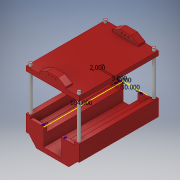
# Autodesk Inventor part: Gondola Shape
Saved by Autodesk Inventor 2018 (Build 220112000, 112)
## iProperties
Created: 2018-01-19
Part Number: Gondola Shape
Material: Steel
Document SubType Name: Modeling
Designer: Joey
Density: 7.85 g/cm^3
Appearance: Red
Author: Joey
Autodesk Inventor part; units mm, degrees
ref_plane "YZ Plane" through (0, 0, 0) normal (1, 0, 0) x (0, 1, 0)
ref_plane "XZ Plane" through (0, 0, 0) normal (0, 1, 0) x (-1, 0, 0)
ref_plane "XY Plane" through (0, 0, 0) normal (0, 0, 1) x (1, 0, 0)
sketch "Sketch1" plane through (0, 0, 0) normal (0, 0, 1) x (1, 0, 0)
  line L0 (0, 3431.8221) -> (1930.4, 3431.8221) construction
  line L1 (1930.4, 3431.8221) -> (1930.4, 0) construction
  line L2 (1930.4, 0) -> (0, 0) construction
  line L3 (0, 0) -> (0, 3431.8221) construction
  line L4 (50.8, 812.8) -> (150.6424, 812.8)
  line L5 (150.6424, 812.8) -> (406.4, 508)
  line L6 (406.4, 508) -> (1524, 508)
  line L7 (1524, 508) -> (1779.7576, 812.8)
  line L8 (1779.7576, 812.8) -> (1879.6, 812.8)
  line L9 (1879.6, 812.8) -> (1879.6, 1371.6)
  line L10 (1879.6, 1371.6) -> (1727.2, 1371.6)
  line L11 (50.8, 1371.6) -> (50.8, 812.8)
  line L12 (203.2, 1371.6) -> (203.2, 1270)
  line L13 (203.2, 1270) -> (660.4, 1270)
  line L14 (660.4, 1270) -> (660.4, 660.4)
  line L15 (660.4, 660.4) -> (1270, 660.4)
  line L16 (1270, 660.4) -> (1270, 1270)
  line L17 (1270, 1270) -> (1727.2, 1270)
  line L18 (1727.2, 1270) -> (1727.2, 1371.6)
  line L19 (203.2, 1371.6) -> (50.8, 1371.6)
  dimension "d9" = 130
  dimension "d27" = 558.8
  dimension "d29" = 1828.8
  dimension "d30" = 1930.4
  dimension "d37" = 101.6
  dimension "d46" = 508
  dimension "d47" = 50.8
  dimension "d51" = 152.4
  dimension "d68" = 1117.6
  dimension "d69" = 304.8
  dimension "d74" = 609.6
  dimension "d77" = 609.6
  constraints: 32 end point, 12 perpendicular, 5 equal length, 4 horizontal, 2 vertical, 1 coincident, 1 collinear, 1 point on line, 2 other
  measures "d9" angle of L5 L4
  measures "d27" distance of L8.end L9.end
  measures "d29" distance between parallel lines of L9 L11
  measures "d30" distance of L1.end L2.end
  measures "d37" distance of L17.end L10.end
  measures "d46" distance from line of L6 point (0, 0)
  measures "d47" distance between parallel lines of L3 L11
  measures "d51" distance of L12.start L11.start
  measures "d68" distance of L5.end L6.end
  measures "d69" distance between parallel lines of L4 L6
  measures "d74" distance of L14.end L15.end
  measures "d77" distance of L13.end L14.end
extrude "Extrusion1" add sketch "Sketch1" along normal mid plane 2743.2
sketch "Sketch2" plane through (203.2, 1270, -1371.6) normal (0, 1, 0) x (1, 0, 0)
  line L0 (0, 0) -> (457.2, 0) construction
  line L1 (0, 0) -> (0, -2743.2) construction
  line L2 (457.2, -2743.2) -> (0, -2743.2) construction
  line L3 (457.2, 0) -> (457.2, -2743.2) construction
  line L4 (1066.8, 0) -> (1524, 0) construction
  line L5 (1066.8, 0) -> (1066.8, -2743.2) construction
  line L6 (1524, -2743.2) -> (1066.8, -2743.2) construction
  line L7 (1524, 0) -> (1524, -2743.2) construction
  line L8 (457.2, -2641.6) -> (0, -2641.6)
  line L9 (0, -2641.6) -> (0, -101.6)
  line L10 (0, -101.6) -> (457.2, -101.6)
  line L11 (457.2, -101.6) -> (457.2, -2641.6)
  line L12 (1066.8, -101.6) -> (1524, -101.6)
  line L13 (1524, -101.6) -> (1524, -2641.6)
  line L14 (1524, -2641.6) -> (1066.8, -2641.6)
  line L15 (1066.8, -2641.6) -> (1066.8, -101.6)
  line L16 (0, 0) -> (0, -2743.2) construction
  line L17 (0, -1371.6) -> (1524, -1371.6) construction
  point P0 (-203.2, -1371.6)
  dimension "d80" = 2540
  constraints: 18 end point, 6 point on line, 4 parallel, 2 horizontal, 2 midpoint, 2 perpendicular, 1 other
  measures "d80" distance between parallel lines of L10 L8
extrude "Extrusion2" cut sketch "Sketch2" against normal blind 203.2
sketch "Sketch4" plane through (0, 0, 0) normal (0, 0, 1) x (1, 0, 0)
  line L0 (0, 3431.8221) -> (1930.4, 3431.8221) construction
  line L1 (1930.4, 3431.8221) -> (1930.4, 0) construction
  line L2 (1930.4, 0) -> (0, 0) construction
  line L3 (0, 0) -> (0, 3431.8221) construction
  line L4 (50.8, 2794) -> (1879.6, 2794)
  line L5 (1879.6, 2794) -> (1879.6, 2641.6)
  line L6 (1879.6, 2641.6) -> (1828.8, 2641.6)
  line L7 (1286.9333, 2641.6) -> (1236.1333, 2641.6)
  line L8 (694.2667, 2641.6) -> (643.4667, 2641.6)
  line L9 (101.6, 2641.6) -> (50.8, 2641.6)
  line L10 (50.8, 2641.6) -> (50.8, 2794)
  arc A0 (643.4667, 2641.6) -> (101.6, 2641.6) centre (372.5333, 2242.2281) ccw construction
  arc A1 (1236.1333, 2641.6) -> (694.2667, 2641.6) centre (965.2, 2242.2281) ccw construction
  arc A2 (1828.8, 2641.6) -> (1286.9333, 2641.6) centre (1557.8667, 2242.2281) ccw construction
  line L11 (1557.8667, 2724.8281) -> (372.5333, 2724.8281) construction
  line L12 (1727.2, 1371.6) -> (1879.6, 1371.6) projected
  line L13 (1524, 508) -> (406.4, 508) projected
  line L14 (50.8, 2641.6) -> (1879.6, 2641.6)
  point P0 (965.2, 2724.8281)
  dimension "d98" = 1930.4
  dimension "d107" = 152.4
  dimension "d109" = 50.8
  dimension "d110" = 482.6
  dimension "d114" = 2286
  dimension "d115" = 50.8
  dimension "d117" = 1828.8
  constraints: 18 end point, 9 point on circle, 6 point on line, 3 centre point, 3 collinear, 3 perpendicular, 2 equal radius, 2 horizontal, 1 coincident, 1 midpoint, 1 parallel, 1 vertical, 2 other
  measures "d98" distance of L1.end L2.end
  measures "d107" distance of L4.end L5.end
  measures "d109" distance of L8.start L8.end
  measures "d110" radius of A1
  measures "d114" distance between parallel lines of L4 L13
  measures "d115" distance between parallel lines of L1 L5
  measures "d117" distance of L4.start L4.end
extrude "Extrusion4" add sketch "Sketch4" along normal mid plane 2743.2
shell "Shell2" thickness 25.4 removed faces 1 at (1270, 2641.6, -457.2)
sketch "Sketch5" plane through (0, 0, 0) normal (0, 0, 1) x (1, 0, 0)
  line L0 (50.8, 2794) -> (1879.6, 2794) construction
  line L1 (508, 2794) -> (1422.4, 2794)
  line L2 (1422.4, 2794) -> (1422.4, 2844.8)
  line L3 (1422.4, 2844.8) -> (1158.4355, 2997.2)
  line L4 (1158.4355, 2997.2) -> (771.9645, 2997.2)
  line L5 (771.9645, 2997.2) -> (508, 2844.8)
  line L6 (508, 2844.8) -> (508, 2794)
  line L7 (965.2, 2794) -> (965.2, 2997.2) construction
  circle A0 centre (965.2, 2921) radius 25.4
  circle A1 centre (850.9, 2921) radius 25.4
  circle A2 centre (1079.5, 2921) radius 25.4
  line L8 (850.9, 2921) -> (1079.5, 2921) construction
  point P0 (0, 0)
  dimension "d118" = 50.8
  dimension "d119" = 203.2
  dimension "d120" = 30
  dimension "d121" = 914.4
  dimension "d122" = 50.8
  dimension "d123" = 76.2
  dimension "d124" = 50.8
  dimension "d125" = 50.8
  dimension "d126" = 114.3
  dimension "d127" = 114.3
  dimension "d128" = 76.2
  constraints: 16 end point, 3 centre point, 2 equal length, 2 horizontal, 2 midpoint, 2 parallel, 1 collinear, 1 perpendicular, 1 point on line, 1 vertical
  measures "d118" distance of L1.end L2.end
  measures "d119" distance between parallel lines of L0 L4
  measures "d120" angle of L5 L0
  measures "d121" distance between parallel lines of L2 L6
  measures "d122" diameter of A0
  measures "d123" distance from line of L4 A0.centre
  measures "d124" diameter of A1
  measures "d125" diameter of A2
  measures "d126" distance of A0.centre L8.end
  measures "d127" distance of A0.centre L8.start
  measures "d128" distance between parallel lines of L8 L4
extrude "Extrusion5" add sketch "Sketch5" along normal mid plane 2743.2
sketch "Sketch6" plane through (1422.4, 2794, 1371.6) normal (1, 0, 0) x (0, 0, -1)
  line L0 (2743.2, 50.8) -> (0, 50.8) construction
  line L1 (0, 0) -> (0, 50.8) construction
  line L2 (2743.2, 0) -> (0, 0) construction
  line L3 (2743.2, 50.8) -> (2743.2, 0) construction
  line L4 (2743.2, 203.2) -> (0, 203.2) construction
  line L5 (0, 50.8) -> (0, 203.2) construction
  line L6 (2743.2, 50.8) -> (0, 50.8) construction
  line L7 (2743.2, 203.2) -> (2743.2, 50.8) construction
  line L8 (0, 0) -> (2743.2, 0) projected
  line L9 (228.6, 203.2) -> (2514.6, 203.2)
  line L10 (2514.6, 203.2) -> (2514.6, 0)
  line L11 (2514.6, 0) -> (228.6, 0)
  line L12 (228.6, 0) -> (228.6, 203.2)
  line L13 (2743.2, 203.2) -> (0, 203.2) projected
  line L14 (1371.6, 203.2) -> (1371.6, 0) construction
  point P0 (1371.6, -2794)
  dimension "d131" = 1143
  constraints: 10 end point, 2 midpoint, 2 parallel, 2 point on line, 1 horizontal, 1 perpendicular, 1 vertical
  measures "d131" distance between parallel lines of L14 L10
extrude "Extrusion6" cut sketch "Sketch6" against normal through all
sketch "Sketch7" plane through (1879.6, 2641.6, 1371.6) normal (1, 0, 0) x (0, 0, -1)
  line L0 (0, 152.4) -> (2743.2, 152.4) construction
  line L1 (0, 0) -> (0, 152.4) construction
  line L2 (0, 0) -> (2743.2, 0) construction
  line L3 (2743.2, 152.4) -> (2743.2, 0) construction
  line L4 (0, 0) -> (50.8, 0)
  line L5 (0, 0) -> (2743.2, 0) construction
  line L6 (897.4667, 0) -> (948.2667, 0)
  line L7 (1794.9333, 0) -> (1845.7333, 0)
  line L8 (2692.4, 0) -> (2743.2, 0)
  arc A0 (897.4667, 0) -> (50.8, 0) centre (474.1333, -231.7146) ccw
  arc A1 (1794.9333, 0) -> (948.2667, 0) centre (1371.6, -231.7146) ccw
  arc A2 (2692.4, 0) -> (1845.7333, 0) centre (2269.0667, -231.7146) ccw
  line L9 (50.8, 0) -> (897.4667, 0)
  line L10 (948.2667, 0) -> (1794.9333, 0)
  line L11 (1845.7333, 0) -> (2692.4, 0)
  line L12 (474.1333, 250.8854) -> (2269.0667, 250.8854) construction
  point P0 (1371.6, -2641.6)
  dimension "d134" = 50.8
  dimension "d138" = 482.6
  constraints: 16 end point, 8 point on circle, 6 collinear, 6 point on line, 3 centre point, 2 equal radius, 2 tangent, 1 horizontal
  measures "d134" distance of L1.start L4.end
  measures "d138" radius of A1
extrude "Extrusion7" [suppressed]
sketch "Sketch9" plane through (0, 0, -1371.6) normal (0, 0, -1) x (-1, 0, 0)
  line L0 (-50.8, 2641.6) -> (-1879.6, 2641.6) construction
  line L1 (-1879.6, 2641.6) -> (-1828.8, 2641.6)
  line L2 (-1286.9333, 2641.6) -> (-1236.1333, 2641.6)
  line L3 (-694.2667, 2641.6) -> (-643.4667, 2641.6)
  line L4 (-50.8, 2641.6) -> (-50.8, 2794) construction
  line L5 (-101.6, 2641.6) -> (-50.8, 2641.6)
  arc A0 (-1286.9333, 2641.6) -> (-1828.8, 2641.6) centre (-1557.8667, 2198.0407) ccw
  arc A1 (-694.2667, 2641.6) -> (-1236.1333, 2641.6) centre (-965.2, 2198.0407) ccw
  arc A2 (-101.6, 2641.6) -> (-643.4667, 2641.6) centre (-372.5333, 2198.0407) ccw
  line L6 (-1828.8, 2641.6) -> (-1286.9333, 2641.6)
  line L7 (-1236.1333, 2641.6) -> (-694.2667, 2641.6)
  line L8 (-643.4667, 2641.6) -> (-101.6, 2641.6)
  line L9 (-1879.6, 2641.6) -> (-1879.6, 2794) projected
  line L10 (-1879.6, 2717.8) -> (-50.8, 2717.8) construction
  line L11 (-50.8, 2794) -> (-50.8, 2641.6) projected
  point P0 (0, 0)
  dimension "d152" = 50.8
  constraints: 16 end point, 6 point on circle, 6 point on line, 5 collinear, 3 centre point, 3 tangent, 2 equal radius, 2 horizontal, 2 midpoint
  measures "d152" distance of L0.end L1.end
extrude "Extrusion9" [suppressed]
sketch "Sketch8" plane through (50.8, 1371.6, 1371.6) normal (0, 1, 0) x (1, 0, 0)
  circle A0 centre (76.2, 2667) radius 50.8
  line L0 (0, 0) -> (0, 2743.2) construction
  line L1 (99.8424, 2743.2) -> (0, 2743.2) construction
  circle A1 centre (1752.6, 2667) radius 50.8
  circle A2 centre (76.2, 76.2) radius 50.8
  circle A3 centre (1752.6, 76.2) radius 50.8
  point P0 (-50.8, 1371.6)
  dimension "d139" = 101.6
  dimension "d140" = 76.2
  dimension "d141" = 76.2
  dimension "d144" = 1676.4
  dimension "d147" = 2590.8
  constraints: 4 centre point, 1 horizontal, 1 vertical, 6 other
  measures "d139" diameter of A0
  measures "d140" distance from line of A0.centre L0
  measures "d141" distance from line of A0.centre L1
  measures "d144" distance of A0.centre A1.centre
  measures "d147" distance of A0.centre A2.centre
extrude "Extrusion8" add sketch "Sketch8" along normal blind 1524
sketch "Sketch10" plane through (203.2, 1270, 1371.6) normal (0, 1, 0) x (1, 0, 0)
  circle A0 centre (381, 2692.4) radius 38.1
  line L0 (457.2, 2743.2) -> (457.2, 0) projected
  line L1 (1320.8, 2743.2) -> (203.2, 2743.2) projected
  circle A1 centre (1143, 2692.4) radius 38.1
  circle A2 centre (381, 50.8) radius 38.1
  circle A3 centre (1143, 50.8) radius 38.1
  point P0 (-203.2, 1371.6)
  dimension "d158" = 76.2
  dimension "d159" = 76.2
  dimension "d160" = 50.8
  dimension "d163" = 762
  dimension "d170" = 2641.6
  constraints: 4 centre point, 1 horizontal, 1 vertical, 6 other
  measures "d158" diameter of A0
  measures "d159" distance from line of A0.centre L0
  measures "d160" distance from line of L1 A0.centre
  measures "d163" distance of A0.centre A1.centre
  measures "d170" distance of A0.centre A2.centre
body "Solid1"
